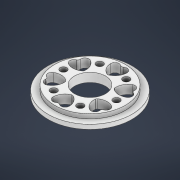
# Autodesk Inventor part: wheelcap
Saved by Autodesk Inventor 2022 (Build 260153000, 153)
## iProperties
Created: 2021-09-22
Part Number: wheelcap
Material: ABS プラスチック
Document SubType Name: Modeling
Designer: shiok
Density: 1.06 g/cm^3
Appearance: 滑らか - 白
Mass: 0.355487 g
Surface Area: 6.92112 cm^2
Volume: 0.335365 cm^3
Author: shiok
Autodesk Inventor part; units mm, degrees
ref_plane "YZ Plane" through (0, 0, 0) normal (1, 0, 0) x (0, 1, 0)
ref_plane "XZ Plane" through (0, 0, 0) normal (0, 1, 0) x (-1, 0, 0)
ref_plane "XY Plane" through (0, 0, 0) normal (0, 0, 1) x (1, 0, 0)
sketch "スケッチ1" plane through (0, 0, 0) normal (0, 1, 0) x (-1, 0, 0)
  circle A0 centre (0, 0) radius 9.5
  dimension "d0" = 19
  constraints: 1 centre point, 1 coincident
  measures "d0" diameter of A0
extrude "押し出し1" add sketch "スケッチ1" along normal blind 1
sketch "スケッチ2" plane through (0, 1, 0) normal (0, 1, 0) x (1, 0, 0)
  circle A0 centre (0, 0) radius 8
  dimension "d4" = 16
  constraints: 1 centre point, 1 coincident
  measures "d4" diameter of A0
extrude "押し出し2" add sketch "スケッチ2" along normal blind 1
sketch "スケッチ4" plane through (0, 2, 0) normal (0, 1, 0) x (1, 0, 0)
  circle A0 centre (0, 0) radius 3.5
  dimension "d20" = 7
  constraints: 1 centre point, 1 coincident
  measures "d20" diameter of A0
extrude "押し出し4" cut sketch "スケッチ4" against normal blind 10
sketch "スケッチ5" plane through (0, 2, 0) normal (0, 1, 0) x (1, 0, 0)
  arc A0 (1.8278, 6.5459) -> (0, 6.6723) centre (0.9095, 6.5459) ccw
  arc A1 (0, 3.9641) -> (1.8278, 6.5459) centre (-0.9095, 6.5459) ccw
  line L0 (0, 6.6723) -> (0, 3.9641)
  line L1 (0.9095, 6.5459) -> (0, 6.5459) construction
  line L2 (-0.9095, 6.5459) -> (0, 6.5459) construction
  line L3 (1.8278, 4.5823) -> (1.8278, 2.8488) construction
  line L4 (1.8278, 5.2864) -> (1.8278, 3.0604) construction
  line L5 (-0.8113, 7.4641) -> (2.8855, 7.4641) construction
  line L6 (1.0371, 7.4641) -> (1.101, 7.9239) construction
  line L7 (0, 3.9641) -> (0, 3.5) construction
  circle A2 centre (0, 0) radius 3.5 construction
  circle A3 centre (0, 0) radius 8 construction
  line L8 (-0.0992, 5.958) -> (0.183, 7.9894) construction
  arc A4 (0, 6.6723) -> (-1.8278, 6.5459) centre (-0.9095, 6.5459) ccw
  arc A5 (-1.8278, 6.5459) -> (0, 3.9641) centre (0.9095, 6.5459) ccw
  circle A6 centre (3, 5.1962) radius 0.75
  circle A7 centre (0, 0) radius 6 construction
  dimension "d33" = 12
  dimension "d24" = 3.5
  dimension "d31" = 1.5
  dimension "d32" = 30
  constraints: 18 end point, 10 point on circle, 8 point on line, 5 centre point, 4 tangent, 2 collinear, 2 equal length, 1 coincident, 1 horizontal, 1 midpoint, 1 parallel, 1 perpendicular, 1 symmetric about line, 1 vertical, 1 vertical alignment, 8 other
  measures "d24" distance from line of L0.end L5
  measures "d31" diameter of A6
extrude "押し出し5" cut sketch "スケッチ5" against normal blind 10
fillet "フィレット1" radius 0.5 2 edges at (0, 1, -6.6723) (0, 1, -3.9641)
pattern_circular "円形状パターン1" count 6 over 360 about axis through (0, -10, 0) along (0, 1, 0) of "押し出し5", "フィレット1"
